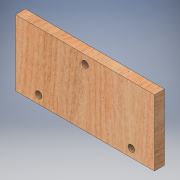
# Autodesk Inventor part: framePlate
Saved by Autodesk Inventor 2016 (Build 200138000, 138)
## iProperties
Created: 2015-09-21
Part Number: framePlate
Material: Generic
Document SubType Name: Modeling
Designer: xdlea
Density: 1 g/cm^3
Appearance: Birch - Natural Polished
Author: xdlea
Autodesk Inventor part; units mm, degrees
ref_plane "YZ Plane" through (0, 0, 0) normal (1, 0, 0) x (0, 1, 0)
ref_plane "XZ Plane" through (0, 0, 0) normal (0, 1, 0) x (-1, 0, 0)
ref_plane "XY Plane" through (0, 0, 0) normal (0, 0, 1) x (1, 0, 0)
sketch "Sketch1" plane through (0, 0, 0) normal (0, 0, 1) x (1, 0, 0)
  line L0 (-133.35, -63.5) -> (133.35, -63.5)
  line L1 (133.35, -63.5) -> (133.35, 63.5)
  line L2 (133.35, 63.5) -> (-133.35, 63.5)
  line L3 (-133.35, 63.5) -> (-133.35, -63.5)
  line L4 (-133.35, -63.5) -> (133.35, 63.5) construction
  line L5 (133.35, -63.5) -> (-133.35, 63.5) construction
  line L6 (0, 88.9) -> (0, -88.9) construction
  circle A0 centre (0, 47.625) radius 6.35
  circle A1 centre (-88.9, -47.625) radius 6.35
  circle A2 centre (88.9, -47.625) radius 6.35
  line L7 (-200.025, 0) -> (200.025, 0) construction
  point P0 (0, 0)
  point P1 (0, 0)
  dimension "d0" = 266.7
  dimension "d1" = 127
  dimension "d9" = 47.625
  dimension "d10" = 47.625
  dimension "d11" = 177.8
  dimension "d12" = 12.7
  constraints: 12 end point, 3 centre point, 3 midpoint, 2 equal radius, 2 parallel, 1 horizontal, 1 horizontal alignment, 1 perpendicular, 1 point on line, 1 other
  measures "d0" distance of L1.end L2.end
  measures "d1" distance of L0.end L1.end
  measures "d9" distance from line of L7 A0.centre
  measures "d10" distance from line of L7 A1.centre
  measures "d11" distance of A2.centre A1.centre
  measures "d12" diameter of A0
extrude "Extrusion2" add sketch "Sketch1" along normal blind 19.05
equation "\"d0\" = Length"
equation "\"d1\" = FrameHeight"
equation "\"d9\" = 0.375 * FrameHeight"
equation "\"d10\" = d9"
equation "\"d11\" = 0.666667 * Length"
equation "\"d7\" = Thickness"
equation "\"FrameHeight\" = 127"
equation "\"Length\" = 266.7"
equation "\"Thickness\" = 19.05"
body "Solid2"
